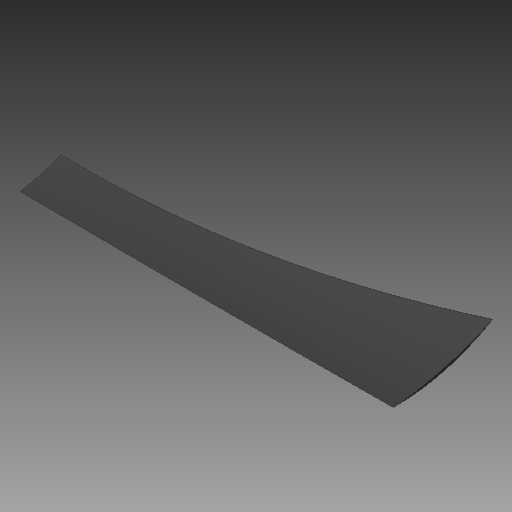
# Autodesk Inventor part: test_front_element_2
Saved by Autodesk Inventor 2018.1 (Build 221171000, 171)
## iProperties
Created: 2017-10-30
Part Number: test_front_element_2
Material: 一般
Document SubType Name: Modeling
Designer: ku_sk
Density: 1 g/cm^3
Appearance: 既定
Author: ku_sk
Autodesk Inventor part; units mm, degrees
ref_plane "XZ Plane" through (0, 0, 0) normal (0, 1, 0) x (-1, 0, 0)
ref_plane "作業平面1" through (150, 0, 0) normal (1, 0, 0) x (0, 1, 0)
ref_plane "作業平面2" through (325, 0, 0) normal (1, 0, 0) x (0, 1, 0)
sketch "スケッチ2" plane through (0, 0, 0) normal (1, 0, 0) x (0, 1, 0)
  arc A0 (0.4022, -2.1485) -> (9.992, -37.9382) centre (251.688, 46.0036) ccw
  arc A1 (0.2045, -2.1776) -> (9.8063, -38.0119) centre (116.8603, 9.8767) ccw
  line L0 (0, -57.2007) -> (0, 63.2044) projected
  line L1 (0, 0) -> (10.718, -40)
  arc A2 (9.8063, -38.0119) -> (9.992, -37.9382) centre (9.8976, -37.9711) ccw
  arc A3 (0.4022, -2.1485) -> (0.2045, -2.1776) centre (0.304, -2.1673) ccw
  dimension "d6" = 40
  dimension "d8" = 15
  dimension "d9" = 0.1
  dimension "d10" = 0.1
  constraints: 12 point on circle, 4 centre point, 4 tangent, 2 end point, 1 coincident
  measures "d6" vertical distance of L1.end L1.start
  measures "d8" angle of L0 L1
  measures "d9" radius of A2
  measures "d10" radius of A3
sketch "スケッチ3" plane through (150, 0, 0) normal (1, 0, 0) x (0, 1, 0)
  line L0 (0, 0) -> (11.5434, -50)
  arc A0 (0.1854, -1.5241) -> (11.0419, -48.5488) centre (234.0668, 27.7061) ccw
  arc A1 (-0.0138, -1.5364) -> (10.8575, -48.6252) centre (106.5896, -1.7244) ccw
  line L1 (0, -65.5412) -> (0, 43.2473) projected
  arc A2 (10.8575, -48.6252) -> (11.0419, -48.5488) centre (10.9473, -48.5812) ccw
  arc A3 (0.1854, -1.5241) -> (-0.0138, -1.5364) centre (0.0862, -1.5365) ccw
  dimension "d11" = 13
  dimension "d12" = 50
  dimension "d13" = 0.1
  constraints: 12 point on circle, 4 centre point, 4 tangent, 2 end point, 1 equal radius
  measures "d11" angle of L1 L0
  measures "d12" vertical distance of L0.start L0.end
  measures "d13" radius of A2
sketch "スケッチ4" plane through (325, 0, 0) normal (1, 0, 0) x (0, 1, 0)
  line L0 (0, 0) -> (24.1154, -90)
  arc A0 (0.1697, -1.9542) -> (23.2853, -88.2227) centre (260.8799, 21.6717) ccw
  arc A1 (-0.0299, -1.9623) -> (23.1084, -88.3155) centre (166.8575, -3.5215) ccw
  line L1 (0, -112.3343) -> (0, 44.0061) projected
  arc A2 (23.1084, -88.3155) -> (23.2853, -88.2227) centre (23.1945, -88.2647) ccw
  arc A3 (0.1697, -1.9542) -> (-0.0299, -1.9623) centre (0.0701, -1.9632) ccw
  dimension "d18" = 15
  dimension "d19" = 90
  dimension "d20" = 0.1
  constraints: 12 point on circle, 4 centre point, 4 tangent, 2 end point, 1 equal radius
  measures "d18" angle of L1 L0
  measures "d19" vertical distance of L0.start L0.end
  measures "d20" radius of A2
loft "ロフト2" add profiles "スケッチ2", "スケッチ3", "スケッチ4"
